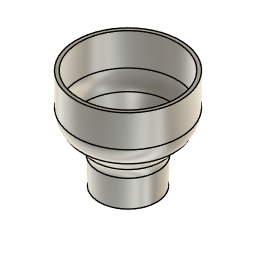
table_saw_dust_extraction_adapter (Autodesk Fusion 360 design; units mm, degrees)
Autodesk Fusion 360 part; units mm, degrees
sketch "Sketch1" plane through (0, 0, 0) normal (0, 0, 1) x (1, 0, 0)
  circle A0 centre (0, 0) radius 17.25
  circle A1 centre (0, 0) radius 15.75
  dimension "d1" = 34.5
  dimension "d4" = -1.5
  constraint coincident A0.centre A1.centre
  measures "d1" diameter of A0
ref_plane "WorkPlane1" through (0, 0, 20) normal (0, 0, 1) x (1, 0, 0)
sketch "Sketch2" plane through (0, 0, 20) normal (0, 0, 1) x (1, 0, 0)
  circle A0 centre (0, 0) radius 17.9
  circle A1 centre (0, 0) radius 16.4
  dimension "d3" = 35.8
  dimension "d5" = -1.5
  constraint coincident A0.centre A1.centre
  measures "d3" diameter of A0
ref_plane "WorkPlane2" through (0, 0, 35) normal (0, 0, 1) x (1, 0, 0)
sketch "Sketch3" plane through (0, 0, 35) normal (0, 0, 1) x (1, 0, 0)
  circle A0 centre (0, 0) radius 29.25
  circle A1 centre (0, 0) radius 31.25
  dimension "d7" = 58.5
  dimension "d8" = 2
  constraint coincident A0.centre A1.centre
  measures "d7" diameter of A0
loft "Loft1" add profiles "Sketch3", "Sketch2" section 1 section 2
loft "Loft2" cut profiles "Sketch3", "Sketch2" section 1 contours A0 section 2 contours A1
loft "Loft3" add profiles "Sketch2", "Sketch1" section 1 section 2
loft "Loft4" cut profiles "Sketch1", "Sketch2" section 1 contours A1 section 2 contours A1
extrude "Extrude1" add sketch "Sketch3" along normal blind 25
fillet "Fillet1" radius 15 2 edges at (-27.2706, 10.5773, 35) (-29.1352, 11.3005, 35)
fillet "Fillet2" radius 10 2 edges at (-16.6887, -6.4729, 20) (-15.2902, -5.9305, 20)
equation "d5 = d4"
